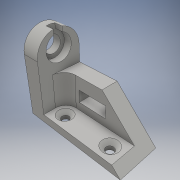
# Autodesk Inventor part: Part1 Drawing
Saved by Autodesk Inventor 2016 (Build 200138000, 138)
## iProperties
Created: 2017-05-22
Part Number: Part1 Drawing
Material: Generic
Document SubType Name: Modeling
Designer: Jaime Sequeira
Density: 1 g/cm^3
Appearance: Default
Author: Jaime Sequeira
Autodesk Inventor part; units mm, degrees
ref_plane "YZ Plane" through (0, 0, 0) normal (1, 0, 0) x (0, 1, 0)
ref_plane "XZ Plane" through (0, 0, 0) normal (0, 1, 0) x (-1, 0, 0)
ref_plane "XY Plane" through (0, 0, 0) normal (0, 0, 1) x (1, 0, 0)
sketch "Sketch1" plane through (0, 0, 0) normal (0, 1, 0) x (-1, 0, 0)
  line L0 (0, 0) -> (-50, 0)
  line L1 (-50, 0) -> (-50, -120)
  line L2 (-50, -120) -> (0, -120)
  line L3 (0, -120) -> (0, 0)
  dimension "d0" = 50
  dimension "d1" = 120
  constraints: 8 end point, 2 parallel, 1 horizontal, 1 perpendicular
  measures "d0" distance of L2.end L1.end
  measures "d1" distance of L1.end L0.end
extrude "Extrusion1" add sketch "Sketch1" along normal blind 10
sketch "Sketch2" plane through (0, 10, 0) normal (0, 1, 0) x (1, 0, 0)
  line L0 (0, 0) -> (50, 0)
  line L1 (50, 0) -> (50, 20)
  line L2 (50, 20) -> (0, 20)
  line L3 (0, 20) -> (0, 0)
  dimension "d4" = 50
  dimension "d5" = 20
  constraints: 8 end point, 2 parallel, 1 horizontal, 1 perpendicular
  measures "d4" distance of L2.end L1.end
  measures "d5" distance of L1.end L0.end
extrude "Extrusion2" add sketch "Sketch2" along normal blind 85
chamfer "Chamfer1" distance 10 angle 45 1 edges at (25, 10, -120)
sketch "Sketch3" plane through (0, 10, 0) normal (0, 1, 0) x (1, 0, 0)
  line L0 (0, 110) -> (0, 20) projected
  line L1 (0, 20) -> (50, 20) projected
  line L2 (0, 110) -> (20, 110)
  line L3 (20, 110) -> (20, 20)
  line L4 (20, 20) -> (0, 20)
  line L5 (0, 20) -> (0, 110)
  point P0 (0, 0)
  dimension "d11" = 20
  constraints: 8 end point, 2 parallel, 1 horizontal, 1 perpendicular, 1 point on line
  measures "d11" distance of L3.end L4.end
extrude "Extrusion3" add sketch "Sketch3" along normal blind 40
chamfer "Chamfer2" distance 40 angle 45 1 edges at (10, 50, -110)
fillet "Fillet1" radius 15 1 edges at (20, 30, -20)
sketch "Sketch4" plane through (50, 95, -20) normal (0, 0, -1) x (-1, 0, 0)
  point P0 (50, -95)
  point P1 (25, -20)
hole "Hole1" at (25, 75, -20) direction (0, 0, 1) diameter 20 depth 20 tip angle 118 counterbore diameter 30 counterbore depth 10
fillet "Fillet2" radius 25 2 edges at (50, 95, -10) (0, 95, -10)
sketch "Sketch5" plane through (0, 10, 0) normal (0, 1, 0) x (1, 0, 0)
  line L0 (35, 35) -> (35, 95)
  point P0 (0, 0)
  dimension "d26" = 60
  constraints: 2 coincident, 2 end point, 1 vertical
  measures "d26" distance of L0.start L0.end
hole "Hole2" at (35, 10, -35) at (35, 10, -95) direction (0, -1, 0) diameter 10 depth 10 tip angle 118 countersink diameter 20 countersink angle 90
sketch "Sketch6" plane through (50, 10, -20) normal (0, 0, -1) x (-1, 0, 0)
  line L0 (20, 79) -> (30, 79)
  line L1 (30, 79) -> (30, 86.8566)
  line L2 (30, 86.8566) -> (20, 86.8566)
  line L3 (20, 86.8566) -> (20, 79)
  point P0 (50, -10)
  constraints: 8 end point, 2 parallel, 1 horizontal, 1 perpendicular
extrude "Extrusion4" cut sketch "Sketch6" against normal blind 10
sketch "Sketch7" plane through (20, 10, -35) normal (1, 0, 0) x (0, 0, -1)
  line L0 (5, 25) -> (40, 25)
  line L1 (40, 25) -> (40, 10)
  line L2 (40, 10) -> (5, 10)
  line L3 (5, 10) -> (5, 25)
  point P0 (-35, -10)
  constraints: 8 end point, 2 parallel, 1 horizontal, 1 perpendicular
extrude "Extrusion5" cut sketch "Sketch7" against normal blind 20
body "Solid1"
